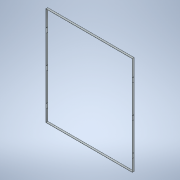
# Autodesk Inventor part: Frame2
Saved by Autodesk Inventor 2021 (Build 250183000, 183)
## iProperties
Created: 2021-07-31
Part Number: Frame2
Material: Zinc
Document SubType Name: Modeling
Designer: Shammy Haider
Density: 7 g/cm^3
Appearance: Zinc
Mass: 8423.52 g
Surface Area: 6930.48 cm^2
Volume: 1203.36 cm^3
Author: Shammy Haider
Autodesk Inventor part; units mm, degrees
ref_plane "YZ Plane" through (0, 0, 0) normal (1, 0, 0) x (0, 1, 0)
ref_plane "XZ Plane" through (0, 0, 0) normal (0, 1, 0) x (-1, 0, 0)
ref_plane "XY Plane" through (0, 0, 0) normal (0, 0, 1) x (1, 0, 0)
sketch "Sketch1" plane through (0, 0, 0) normal (0, 0, 1) x (1, 0, 0)
  line L0 (920, -1050) -> (-920, -1050)
  line L1 (-920, -1050) -> (-920, 1050)
  line L2 (-920, 1050) -> (920, 1050)
  line L3 (920, 1050) -> (920, -1050)
  line L4 (920, -1050) -> (-920, 1050) construction
  line L5 (-920, -1050) -> (920, 1050) construction
  line L6 (924, 1054) -> (-924, 1054)
  line L7 (-924, 1054) -> (-924, -1054)
  line L8 (-924, -1054) -> (924, -1054)
  line L9 (924, -1054) -> (924, 1054)
  point P0 (0, 0)
  dimension "d0" = 1840
  dimension "d1" = 2100
  dimension "d2" = 4
  constraints: 20 end point, 4 parallel, 2 midpoint, 2 perpendicular, 1 horizontal, 3 other
  measures "d0" distance of L1.end L2.end
  measures "d1" distance of L0.end L1.end
  measures "d2" distance between parallel lines of L2 L6
extrude "Extrusion1" add sketch "Sketch1" along normal mid plane 40
sketch "Sketch2" plane through (-920, -1050, 20) normal (1, 0, 0) x (0, 0, -1)
  line L0 (0, 2104) -> (0, -4) projected
  line L1 (40, -4) -> (40, 2104) projected
  line L2 (0, 1750) -> (40, 1750)
  line L3 (40, 1750) -> (40, 1650)
  line L4 (40, 1650) -> (0, 1650)
  line L5 (0, 1650) -> (0, 1750)
  line L6 (0, 2104) -> (40, 2104) projected
  line L7 (0, 1050) -> (40, 1050)
  line L8 (40, 1050) -> (40, 950)
  line L9 (0, 950) -> (0, 1050)
  line L10 (40, 950) -> (0, 950)
  line L11 (0, 350) -> (40, 350)
  line L12 (40, 350) -> (40, 250)
  line L13 (0, 250) -> (0, 350)
  line L14 (40, 250) -> (0, 250)
  line L15 (40, 2100) -> (0, 2100) projected
  point P0 (20, 1050)
  point P1 (0, 250)
  point P2 (40, 350)
  point P3 (0, 950)
  point P4 (40, 1050)
  point P5 (0, 1650)
  point P6 (40, 1750)
  dimension "d5" = 100
  dimension "d9" = 700
  dimension "d24" = 350
  constraints: 24 end point, 2 parallel, 2 point on line, 1 horizontal, 1 perpendicular, 1 vertical, 16 other
  measures "d5" distance between parallel lines of L4 L2
  measures "d9" distance of L2.start L7.start
  measures "d24" distance between parallel lines of L15 L2
extrude "Extrusion2" cut sketch "Sketch2" against normal blind 2.5 contours L2 L1 L4 L0 | L7 L1 L10 L0 | L11 L1 L14 L0
mirror "Mirror1" about plane through (0, 0, 0) normal (1, 0, 0) of "Extrusion2"
sketch "Sketch3" plane through (-922.5, -1050, 20) normal (1, 0, 0) x (0, 0, -1)
  circle A0 centre (20, 340) radius 4
  line L0 (0, 2104) -> (0, -4) projected
  line L1 (0, 350) -> (40, 350) projected
  point P0 (20, 1050)
  dimension "d16" = 8
  dimension "d17" = 20
  dimension "d18" = 10
  constraints: 1 centre point
  measures "d16" diameter of A0
  measures "d17" distance from line of L0 A0.centre
  measures "d18" distance from line of L1 A0.centre
extrude "Extrusion3" cut sketch "Sketch3" against normal blind 1
pattern_linear "Rectangular Pattern1" count 3 spacing 700 along (0, 1, 0) of "Extrusion3"
mirror "Mirror2" about plane through (0, 0, 0) normal (1, 0, 0) of "Extrusion3", "Rectangular Pattern1"
body "Solid1"
